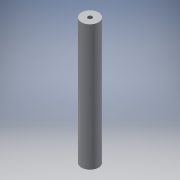
# Autodesk Inventor part: dipoleDiscSpacer_B
Saved by Autodesk Inventor 2016 (Build 200138000, 138)
## iProperties
Company: HERA Project
Created: 2013-06-03
Part Number: dipoleDiscSpacer_B
Material: Acetal Resin, White
Document SubType Name: Modeling
Designer: Rich Bradley
Density: 1.425 g/cm^3
Description: Feed disk spacer
Mass: 26.3641 g
Surface Area: 60.8049 cm^2
Volume: 18.5012 cm^3
Appearance: Smooth - White
Author: David DeBoer
Title: Feed spacer
Autodesk Inventor part; units mm, degrees
ref_plane "YZ Plane" through (0, 0, 0) normal (1, 0, 0) x (0, 1, 0)
ref_plane "XZ Plane" through (0, 0, 0) normal (0, 1, 0) x (-1, 0, 0)
ref_plane "XY Plane" through (0, 0, 0) normal (0, 0, 1) x (1, 0, 0)
sketch "Sketch1" plane through (0, 0, 0) normal (0, 1, 0) x (-1, 0, 0)
  circle A0 centre (0, 0) radius 10
  dimension "d0" = 20
  constraints: 1 centre point, 1 coincident
  measures "d0" diameter of A0
extrude "Extrusion1" add sketch "Sketch1" along normal blind 146.05
sketch "Sketch2" plane through (0, 146.05, 0) normal (0, 1, 0) x (1, 0, 0)
  circle A0 centre (0, 0) radius 10 projected
  circle A1 centre (0, 0) radius 1.7528
  constraints: 1 centre point, 1 coincident
hole "Hole1" at (0, 146.05, 0) direction (0, -1, 0) diameter 4.9276 depth 25 tip angle 118
sketch "Sketch3" plane through (0, 0, 0) normal (0, -1, 0) x (1, 0, 0)
  circle A0 centre (0, 0) radius 10 projected
  circle A1 centre (0, 0) radius 2.7242
  constraints: 1 centre point, 1 coincident
hole "Hole2" at (0, 0, 0) direction (0, 1, 0) diameter 4.9276 depth 25 tip angle 118
body "Solid1"
